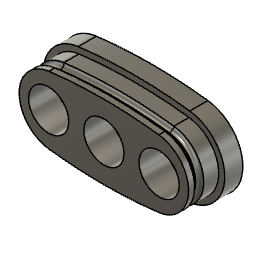
HV Connector Shroud 35mm v3 (Autodesk Fusion 360 design; units mm, degrees)
Autodesk Fusion 360 part; units mm, degrees
sketch "Sketch1" plane through (0, 0, 0) normal (0, 0, 1) x (1, 0, 0) in component "Plug"
  line L0 (-59.9866, -0.0399) -> (-19.4866, -0.0399) construction
  line L1 (-39.7366, -0.0399) -> (-39.7366, 14.7101) construction
  line L2 (-39.7366, -0.0399) -> (-39.7366, -14.7899) construction
  arc A0 (-17.8262, 13.3576) -> (-61.6469, 13.3576) centre (-39.7366, -163.4399) ccw
  arc A1 (-61.6469, -13.4374) -> (-17.8262, -13.4374) centre (-39.7366, 163.3601) ccw
  arc A2 (-17.8262, -13.4374) -> (-17.8262, 13.3576) centre (-19.4866, -0.0399) ccw
  arc A3 (-61.6469, 13.3576) -> (-61.6469, -13.4374) centre (-59.9866, -0.0399) ccw
  dimension "d1" = 27
  dimension "d2" = 27
  dimension "d3" = 40.5
  dimension "d4" = 14.75
  constraint coincident L0.start A3.centre
  constraint coincident L0.end A2.centre
  constraint horizontal L0
  constraint midpoint L0 L1.start
  constraint perpendicular L0 L1
  constraint symmetric L0 L1.start L2.start
  constraint symmetric L0 L1.end L2.end
  constraint coincident L1.end A0
  constraint tangent A0 A2
  constraint tangent A0 A3
  constraint symmetric L0 A0.end A1.start
  constraint symmetric L0 A0.start A1.end
  constraint symmetric L0 A0 A1
  measures "d1" diameter of A2
  measures "d2" diameter of A3
  measures "d3" distance of L0.end L0.start
  measures "d4" distance of L1.start L1.end
extrude "Extrude1" add sketch "Sketch1" along normal blind 2.4 makes body 1 in component "Plug"
sketch "Sketch2" plane through (0, 0, 0) normal (0, 0, 1) x (1, 0, 0) in component "Plug"
sketch "Sketch3" plane through (0, 0, 2.4) normal (0, 0, 1) x (1, 0, 0) in component "Plug"
  arc A0 (-61.6469, 13.3576) -> (-61.6469, -13.4374) centre (-59.9866, -0.0399) ccw
  arc A1 (-61.6469, -13.4374) -> (-17.8262, -13.4374) centre (-39.7366, 163.3601) ccw
  arc A2 (-17.8262, -13.4374) -> (-17.8262, 13.3576) centre (-19.4866, -0.0399) ccw
  arc A3 (-17.8262, 13.3576) -> (-61.6469, 13.3576) centre (-39.7366, -163.4399) ccw
  arc A4 (-61.4501, -11.8495) -> (-18.023, -11.8495) centre (-39.7366, 163.3601) ccw
  arc A5 (-18.023, -11.8495) -> (-18.023, 11.7698) centre (-19.4866, -0.0399) ccw
  arc A6 (-18.023, 11.7698) -> (-61.4501, 11.7698) centre (-39.7366, -163.4399) ccw
  arc A7 (-61.4501, 11.7698) -> (-61.4501, -11.8495) centre (-59.9866, -0.0399) ccw
  dimension "d7" = -1.6
extrude "Extrude2" add sketch "Sketch3" along normal blind 3.6 contours A4 A5 A6 A7 bodies 1 in component "Plug"
sketch "Sketch4" plane through (0, 0, 6) normal (0, 0, 1) x (1, 0, 0) in component "Plug"
  arc A0 (-61.4501, 11.7698) -> (-61.4501, -11.8495) centre (-59.9866, -0.0399) ccw
  arc A1 (-61.4501, -11.8495) -> (-18.023, -11.8495) centre (-39.7366, 163.3601) ccw
  arc A2 (-18.023, -11.8495) -> (-18.023, 11.7698) centre (-19.4866, -0.0399) ccw
  arc A3 (-18.023, 11.7698) -> (-61.4501, 11.7698) centre (-39.7366, -163.4399) ccw
  arc A4 (-61.6469, 13.3576) -> (-61.6469, -13.4374) centre (-59.9866, -0.0399) ccw
  arc A5 (-61.6469, -13.4374) -> (-17.8262, -13.4374) centre (-39.7366, 163.3601) ccw
  arc A6 (-17.8262, -13.4374) -> (-17.8262, 13.3576) centre (-19.4866, -0.0399) ccw
  arc A7 (-17.8262, 13.3576) -> (-61.6469, 13.3576) centre (-39.7366, -163.4399) ccw
  dimension "d10" = 1.6
extrude "Extrude3" add sketch "Sketch4" along normal blind 2.4 contours A0 A1 A2 A3 | A4 A5 A6 A7 bodies 1 in component "Plug"
fillet "Fillet1" radius 1.6 8 edges at (-71.8866, -0.0399, 2.4) (-39.7366, 13.1101, 2.4) (-7.5866, -0.0399, 2.4) (-39.7366, -13.1899, 2.4) (-71.8866, -0.0399, 6) (-39.7366, -13.1899, 6) (-7.5866, -0.0399, 6) (-39.7366, 13.1101, 6) on bodies 1 in component "Plug"
sketch "Sketch5" plane through (0, 0, 8.4) normal (0, 0, 1) x (1, 0, 0) in component "Plug"
  arc A0 (-17.8262, 13.3576) -> (-61.6469, 13.3576) centre (-39.7366, -163.4399) ccw
  arc A1 (-61.6469, 13.3576) -> (-61.6469, -13.4374) centre (-59.9866, -0.0399) ccw
  arc A2 (-61.6469, -13.4374) -> (-17.8262, -13.4374) centre (-39.7366, 163.3601) ccw
  arc A3 (-17.8262, -13.4374) -> (-17.8262, 13.3576) centre (-19.4866, -0.0399) ccw
  line L0 (-5.9866, -0.0399) -> (-73.4866, -0.0399) construction
  circle A4 centre (-61.7366, -0.0399) radius 6.5
  circle A5 centre (-39.7366, -0.0399) radius 6.5
  circle A6 centre (-17.7366, -0.0399) radius 6.5
  dimension "d14" = 13
  dimension "d15" = 13
  dimension "d16" = 13
  dimension "d17" = 22
  dimension "d18" = 22
  constraint midpoint A3 L0.start
  constraint midpoint A1 L0.end
  constraint coincident L0 A5.centre
  constraint coincident L0 A6.centre
  constraint midpoint L0 A5.centre
  measures "d14" diameter of A4
  measures "d15" diameter of A5
  measures "d16" diameter of A6
  measures "d17" distance of A5.centre A6.centre
  measures "d18" distance of A4.centre A5.centre
extrude "Extrude4" cut sketch "Sketch5" against normal blind 8.4 contours A4 | A5 | A6 bodies 1 in component "Plug"
sketch "Sketch6" plane through (0, 0, 0) normal (0, 0, -1) x (-1, 0, 0) in component "Plug"
  circle A0 centre (61.7366, -0.0399) radius 6.5
  circle A1 centre (39.7366, -0.0399) radius 6.5
  circle A2 centre (17.7366, -0.0399) radius 6.5
  arc A3 (61.6469, -13.4374) -> (61.6469, 13.3576) centre (59.9866, -0.0399) ccw
  arc A4 (61.6469, 13.3576) -> (17.8262, 13.3576) centre (39.7366, -163.4399) ccw
  arc A5 (17.8262, 13.3576) -> (17.8262, -13.4374) centre (19.4866, -0.0399) ccw
  arc A6 (17.8262, -13.4374) -> (61.6469, -13.4374) centre (39.7366, 163.3601) ccw
  circle A7 centre (17.7366, -0.0399) radius 8.3
  circle A8 centre (39.7366, -0.0399) radius 8.3
  circle A9 centre (61.7366, -0.0399) radius 8.3
  arc A10 (18.1214, -11.0556) -> (61.3518, -11.0556) centre (39.7366, 163.3601) ccw
  arc A11 (61.3518, -11.0556) -> (61.3518, 10.9758) centre (59.9866, -0.0399) ccw
  arc A12 (61.3518, 10.9758) -> (18.1214, 10.9758) centre (39.7366, -163.4399) ccw
  arc A13 (18.1214, 10.9758) -> (18.1214, -11.0556) centre (19.4866, -0.0399) ccw
  dimension "d21" = 1.8
  dimension "d22" = 1.8
  dimension "d23" = 1.8
  dimension "d26" = -2.4
extrude "Extrude5" add sketch "Sketch6" along normal blind 6 bodies 1 in component "Plug"
extrude "Extrude6" add 1 faces at (-49.477, 7.1443, 0) along direction (0, 0, -1) blind 6 on bodies 1 bodies 1 in component "Plug"
sketch "Sketch7" plane through (0, 0, -6) normal (0, 0, -1) x (-1, 0, 0) in component "Plug"
  circle A0 centre (61.7366, -0.0399) radius 6.5
  arc A1 (17.8262, -13.4374) -> (61.6469, -13.4374) centre (39.7366, 163.3601) ccw
  arc A2 (61.6469, -13.4374) -> (61.6469, 13.3576) centre (59.9866, -0.0399) ccw
  arc A3 (61.6469, 13.3576) -> (17.8262, 13.3576) centre (39.7366, -163.4399) ccw
  arc A4 (17.8262, 13.3576) -> (17.8262, -13.4374) centre (19.4866, -0.0399) ccw
  circle A5 centre (17.7366, -0.0399) radius 6.5
  circle A6 centre (39.7366, -0.0399) radius 6.5
  arc A7 (17.5311, -15.8192) -> (61.9421, -15.8192) centre (39.7366, 163.3601) ccw
  arc A8 (61.9421, -15.8192) -> (61.9421, 15.7394) centre (59.9866, -0.0399) ccw
  arc A9 (61.9421, 15.7394) -> (17.5311, 15.7394) centre (39.7366, -163.4399) ccw
  arc A10 (17.5311, 15.7394) -> (17.5311, -15.8192) centre (19.4866, -0.0399) ccw
  circle A11 centre (17.7366, -0.0399) radius 8.3
  circle A12 centre (39.7366, -0.0399) radius 8.3
  circle A13 centre (61.7366, -0.0399) radius 8.3
  dimension "d29" = 2.4
extrude "Extrude7" add sketch "Sketch7" along normal blind 6 separate body makes body 2 at (-26.0263, -0.4536, -10) makes body 3 at (-70.0263, -0.4536, -10) makes body 4 at (-48.0263, -0.4536, -10) makes body 5 at (-56.9147, -15.4313, -6) in component "Plug"
extrude "Extrude8" add 1 faces at (-56.9147, -15.4313, -6) along direction (0, 0, 1) blind 2.4 on bodies 5 bodies 5 2 3 4 1 in component "Plug"
sketch "Sketch8" plane through (0, 0, -12) normal (0, 0, -1) x (-1, 0, 0) in component "Plug"
  circle A0 centre (17.7366, -0.0399) radius 6.5
  circle A1 centre (17.7366, -0.0399) radius 8.3
  circle A2 centre (39.7366, -0.0399) radius 6.5
  circle A3 centre (39.7366, -0.0399) radius 8.3
  circle A4 centre (61.7366, -0.0399) radius 6.5
  circle A5 centre (61.7366, -0.0399) radius 8.3
  circle A6 centre (61.7366, -0.0399) radius 8.5
  circle A7 centre (39.7366, -0.0399) radius 8.5
  circle A8 centre (17.7366, -0.0399) radius 8.5
  dimension "d34" = 0.2
  dimension "d35" = 0.2
  dimension "d36" = 0.2
extrude "Extrude9" add sketch "Sketch8" against normal blind 0.8 contours A6 | A7 | A8 bodies 2 3 4 5 in component "Plug"
fillet "Fillet2" radius 0.2 6 edges at (-9.8118, -3.1136, -12) (-9.9983, 2.9615, -11.2) (-53.8118, -3.1136, -12) (-53.8118, 3.0338, -11.2) (-31.8118, -3.1136, -12) (-31.8118, 3.0338, -11.2) on bodies 2 3 4 in component "Plug"
extrude "Extrude10" cut 1 faces at (-56.9147, -15.4313, -12) along direction (0, 0, 1) blind 3.6 on bodies 5 bodies 5 in component "Plug"
sketch "Sketch1 (2)" plane through (0, 0, -6) normal (0, 0, -1) x (-1, 0, 0)
  circle A0 centre (61.7366, -0.0399) radius 6.5
  arc A1 (17.8262, -13.4374) -> (61.6469, -13.4374) centre (39.7366, 163.3601) ccw
  arc A2 (61.6469, -13.4374) -> (61.6469, 13.3576) centre (59.9866, -0.0399) ccw
  arc A3 (61.6469, 13.3576) -> (17.8262, 13.3576) centre (39.7366, -163.4399) ccw
  arc A4 (17.8262, 13.3576) -> (17.8262, -13.4374) centre (19.4866, -0.0399) ccw
  circle A5 centre (17.7366, -0.0399) radius 6.5
  circle A6 centre (39.7366, -0.0399) radius 6.5
  circle A7 centre (17.7366, -0.0399) radius 8
  circle A8 centre (39.7366, -0.0399) radius 8
  circle A9 centre (61.7366, -0.0399) radius 8
  dimension "d44" = 16
  dimension "d45" = 16
  dimension "d46" = 16
  constraint concentric A5 A7
  constraint concentric A6 A8
  constraint concentric A0 A9
  measures "d44" diameter of A7
  measures "d45" diameter of A8
  measures "d46" diameter of A9
extrude "Extrude11" cut sketch "Sketch1 (2)" against normal blind 14.4 contours A7 | A8 | A9 bodies 5 in component "Plug"
extrude "Extrude12" add 1 faces at (-29.9633, 8.4542, -6) along direction (0, 0, -1) blind 6 on bodies 5 bodies 5 2 3 4 in component "Plug"
extrude "Extrude13" add 1 faces at (-56.9147, -15.4313, -8.4) along direction (0, 0, -1) blind 3.6 on bodies 5 bodies 5 in component "Plug"
extrude "Extrude14" cut 1 faces at (-39.8985, 13.4524, -12) along direction (0, 0, 1) blind 4.8 on bodies 5 bodies 5 in component "Plug"
extrude "Extrude15" add sketch "Sketch6" against normal blind 8.4 contours A7 | A8 | A9 bodies 5 in component "Plug"
extrude "Extrude16" add 3 faces at (-69.2068, -0.4373, -6) (-47.1826, -0.7603, -6) (-25.2068, -0.4373, -6) along direction (0, 0, 1) blind 14.4 on bodies 5 bodies 5 in component "Plug"
sketch "Sketch2 (2)" plane through (0, 0, -7.2) normal (0, 0, -1) x (-1, 0, 0)
  arc A0 (17.5311, 15.7394) -> (17.5311, -15.8192) centre (19.4866, -0.0399) ccw
  arc A1 (17.5311, -15.8192) -> (61.9421, -15.8192) centre (39.7366, 163.3601) ccw
  arc A2 (61.9421, -15.8192) -> (61.9421, 15.7394) centre (59.9866, -0.0399) ccw
  arc A3 (61.9421, 15.7394) -> (17.5311, 15.7394) centre (39.7366, -163.4399) ccw
  circle A4 centre (39.7366, -0.0399) radius 6.5
  circle A5 centre (61.7366, -0.0399) radius 6.5
  circle A6 centre (17.7366, -0.0399) radius 6.5
  circle A7 centre (17.7366, -0.0399) radius 8
  circle A8 centre (39.7366, -0.0399) radius 8
  circle A9 centre (61.7366, -0.0399) radius 8
  dimension "d59" = 16
  dimension "d60" = 16
  dimension "d61" = 16
  constraint concentric A6 A7
  constraint concentric A4 A8
  constraint concentric A5 A9
  measures "d59" diameter of A7
  measures "d60" diameter of A8
  measures "d61" diameter of A9
extrude "Extrude17" cut sketch "Sketch2 (2)" against normal blind 15.6 contours A7 | A8 | A9 bodies 5 in component "Plug"
sketch "Sketch3 (2)" plane through (0, 0, -7.2) normal (0, 0, -1) x (-1, 0, 0)
  circle A0 centre (61.7366, -0.0399) radius 8
  circle A1 centre (39.7366, -0.0399) radius 8
  circle A2 centre (17.7366, -0.0399) radius 8
  arc A3 (17.5311, 15.7394) -> (17.5311, -15.8192) centre (19.4866, -0.0399) ccw
  arc A4 (17.5311, -15.8192) -> (61.9421, -15.8192) centre (39.7366, 163.3601) ccw
  arc A5 (61.9421, -15.8192) -> (61.9421, 15.7394) centre (59.9866, -0.0399) ccw
  arc A6 (61.9421, 15.7394) -> (17.5311, 15.7394) centre (39.7366, -163.4399) ccw
  circle A7 centre (17.7366, -0.0399) radius 10.7
  circle A8 centre (39.7366, -0.0399) radius 10.7
  circle A9 centre (61.7366, -0.0399) radius 10.7
  dimension "d64" = 21.4
  dimension "d65" = 21.4
  dimension "d66" = 21.4
  constraint concentric A2 A7
  constraint concentric A1 A8
  constraint concentric A0 A9
  measures "d64" diameter of A7
  measures "d65" diameter of A8
  measures "d66" diameter of A9
extrude "Extrude18" add sketch "Sketch3 (2)" along normal blind 2.4 contours A3 A4 A5 A6 bodies 5 in component "Plug"
sketch "Sketch4 (2)" plane through (0, 0, -9.6) normal (0, 0, -1) x (-1, 0, 0)
  circle A0 centre (61.7366, -0.0399) radius 10.7
  circle A1 centre (39.7366, -0.0399) radius 10.7
  circle A2 centre (17.7366, -0.0399) radius 10.7
  arc A3 (61.9421, 15.7394) -> (17.5311, 15.7394) centre (39.7366, -163.4399) ccw
  arc A4 (17.5311, 15.7394) -> (17.5311, -15.8192) centre (19.4866, -0.0399) ccw
  arc A5 (17.5311, -15.8192) -> (61.9421, -15.8192) centre (39.7366, 163.3601) ccw
  arc A6 (61.9421, -15.8192) -> (61.9421, 15.7394) centre (59.9866, -0.0399) ccw
  circle A7 centre (17.7366, -0.0399) radius 10.1
  circle A8 centre (39.7366, -0.0399) radius 10.1
  circle A9 centre (61.7366, -0.0399) radius 10.1
  dimension "d69" = -0.6
  dimension "d70" = -0.6
  dimension "d71" = -0.6
extrude "Extrude19" add sketch "Sketch4 (2)" along normal blind 1.2 contours A0 | A1 | A2 | A3 A4 A5 A6 bodies 5 in component "Plug"
fillet "Fillet3" radius 5 3 edges at (-10.278, 2.853, -7.2) (-32.278, 2.853, -7.2) (-54.278, 2.853, -7.2) on bodies 5 in component "Plug"
component "Plug" placed x (1, 0, 0) y (0, 1, 0) z (0, 0, 1) at (0, 0, 0)
component "Cover" placed x (1, 0, 0) y (0, 1, 0) z (0, 0, 1) at (0, 0, 0)
equation "d3 = 67.5 mm - 27 mm"
equation "d4 = ( 29.5 / 2 ) * 1 mm"
equation "d7 = ( -3.2 / 2 ) * 1 mm"
equation "d18 = d17"
equation "d21 = ( ( 16.6 - 13 ) / 2 ) * 1 mm"
equation "d22 = d21"
equation "d23 = d21"
equation "d53 = -8.40 mm + 3.6 mm"
